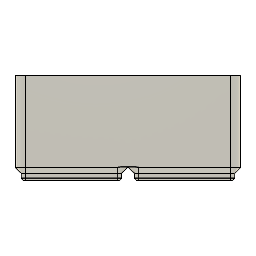
Dupont Jumper Wire (15 cm) (Autodesk Fusion 360 design; units mm, degrees)
Autodesk Fusion 360 part; units mm, degrees
(part 1 of 2)
ref_plane "WorkPlane1" through (0, 0, 0) normal (0, 0, 1) x (1, 0, 0) in component "Gridfinity bin 5x2x5"
sketch "Base plate sketch" plane through (0, 0, 0) normal (0, 0, 1) x (1, 0, 0) in component "Gridfinity bin 5x2x5"
  line L0 (-0.25, -0.25) -> (41.75, -0.25)
  line L1 (41.75, -0.25) -> (41.75, 41.75)
  line L2 (41.75, 41.75) -> (-0.25, 41.75)
  line L3 (-0.25, 41.75) -> (-0.25, -0.25)
  dimension "d326" = 0.25
  dimension "d327" = 0.25
  dimension "d328" = 42
  dimension "d329" = 42
  constraint horizontal L0
  constraint vertical L1
  constraint horizontal L2
  constraint vertical L3
  measures "d326" vertical distance of origin L0.start
  measures "d327" horizontal distance of origin L2.end
  measures "d328" horizontal distance of L0.start L0.end
  measures "d329" vertical distance of L0.end L1.end
extrude "Base top section extrude" add sketch "Base plate sketch" against normal blind 2.4 makes body 1 in component "Gridfinity bin 5x2x5"
fillet "Base corner fillet" radius 4 8 edges at (-0.25, -0.25, -1.2) (41.75, -0.25, -1.2) (41.75, -0.25, -1.2) (41.75, 41.75, -1.2) (41.75, 41.75, -1.2) (-0.25, 41.75, -1.2) (-0.25, 41.75, -1.2) (-0.25, -0.25, -1.2) on bodies 1 in component "Gridfinity bin 5x2x5"
chamfer "Chamfer1" distance 2.4 angle 45 8 edges at (0.9216, 40.5784, -2.4) (-0.25, 20.75, -2.4) (0.9216, 0.9216, -2.4) (20.75, -0.25, -2.4) (40.5784, 0.9216, -2.4) (41.75, 20.75, -2.4) (40.5784, 40.5784, -2.4) (20.75, 41.75, -2.4) on bodies 1 in component "Gridfinity bin 5x2x5"
extrude "Extrude2" add 1 faces at (15.6168, 15.0833, -2.4) along direction (0, 0, -1) blind 2.6 on bodies 1 bodies 1 in component "Gridfinity bin 5x2x5"
chamfer "Chamfer2" distance 0.8 angle 45 8 edges at (2.6186, 38.8814, -5) (20.75, 39.35, -5) (38.8814, 38.8814, -5) (39.35, 20.75, -5) (38.8814, 2.6186, -5) (20.75, 2.15, -5) (2.6186, 2.6186, -5) (2.15, 20.75, -5) on bodies 1 in component "Gridfinity bin 5x2x5"
pattern_linear "R-Pattern1" count 2 spacing 42 along (1, 0, 0) count 5 spacing 42 along (0, 1, 0) of bodies 1 makes body 2 at (68.4167, 16.4167, 0) makes body 3 at (26.4167, 55.75, 0) makes body 4 at (54.4167, 55.75, 0) makes body 5 at (26.4167, 97.75, 0) makes body 6 at (54.4167, 97.75, 0) makes body 7 at (26.4167, 139.75, 0) makes body 8 at (69.75, 141.0833, 0) makes body 9 at (26.4167, 181.75, 0) makes body 10 at (69.75, 183.0833, 0) in component "Gridfinity bin 5x2x5"
sketch "Simple box sketch" plane through (0, 0, 0) normal (0, 0, 1) x (1, 0, 0) in component "Gridfinity bin 5x2x5"
  line L0 (0, 0) -> (83.5, 0)
  line L1 (83.5, 0) -> (83.5, 209.5)
  line L2 (83.5, 209.5) -> (0, 209.5)
  line L3 (0, 209.5) -> (0, 0)
  dimension "d342" = 83.5
  dimension "d343" = 209.5
  constraint horizontal L0
  constraint vertical L1
  constraint horizontal L2
  constraint vertical L3
  constraint coincident L0.start L3
  constraint coincident L3.end L0
  measures "d342" horizontal distance of L0.start L0.end
  measures "d343" vertical distance of L0.end L1.end
extrude "Simple box extrude" add sketch "Simple box sketch" along normal blind 30 separate body makes body 11 in component "Gridfinity bin 5x2x5"
fillet "Bin body corner fillets" radius 3.75 8 edges at (0, 209.5, 15) (83.5, 209.5, 15) (83.5, 209.5, 15) (83.5, 0, 15) (83.5, 0, 15) (0, 0, 15) (0, 0, 15) (0, 209.5, 15) on bodies 11 in component "Gridfinity bin 5x2x5"
ref_plane "WorkPlane2" through (0, 0, 30) normal (0, 0, 1) x (1, 0, 0) in component "Gridfinity bin 5x2x5"
sketch "Simple box at point sketch" plane through (0, 0, 30) normal (0, 0, 1) x (1, 0, 0) in component "Gridfinity bin 5x2x5"
  line L0 (0, 0) -> (83.5, 0)
  line L1 (83.5, 0) -> (83.5, 209.5)
  line L2 (83.5, 209.5) -> (0, 209.5)
  line L3 (0, 209.5) -> (0, 0)
  dimension "d349" = 83.5
  dimension "d350" = 209.5
  constraint horizontal L0
  constraint vertical L1
  constraint horizontal L2
  constraint vertical L3
  constraint coincident L0.start L3
  constraint coincident L3.end L0
  measures "d349" horizontal distance of L0.start L0.end
  measures "d350" vertical distance of L0.end L1.end
extrude "Simple box at point extrude" add sketch "Simple box at point sketch" along normal blind 4.4 separate body makes body 12 in component "Gridfinity bin 5x2x5"
fillet "Lip body corner fillets" radius 3.75 8 edges at (0, 209.5, 32.2) (83.5, 209.5, 32.2) (83.5, 209.5, 32.2) (83.5, 0, 32.2) (83.5, 0, 32.2) (0, 0, 32.2) (0, 0, 32.2) (0, 209.5, 32.2) on bodies 12 in component "Gridfinity bin 5x2x5"
ref_plane "WorkPlane3" through (0, 0, 35) normal (0, 0, 1) x (1, 0, 0) in component "Gridfinity bin 5x2x5"
sketch "Base plate sketch (1)" plane through (0, 0, 35) normal (0, 0, 1) x (1, 0, 0) in component "Gridfinity bin 5x2x5"
  line L0 (-0.5, -0.5) -> (84, -0.5)
  line L1 (84, -0.5) -> (84, 210)
  line L2 (84, 210) -> (-0.5, 210)
  line L3 (-0.5, 210) -> (-0.5, -0.5)
  dimension "d356" = 0.5
  dimension "d357" = 0.5
  dimension "d358" = 84.5
  dimension "d359" = 210.5
  constraint horizontal L0
  constraint vertical L1
  constraint horizontal L2
  constraint vertical L3
  measures "d356" vertical distance of origin L0.start
  measures "d357" horizontal distance of origin L2.end
  measures "d358" horizontal distance of L0.start L0.end
  measures "d359" vertical distance of L0.end L1.end
extrude "Base top section extrude (1)" add sketch "Base plate sketch (1)" against normal blind 2.4 separate body makes body 13 in component "Gridfinity bin 5x2x5"
fillet "Base corner fillet (1)" radius 4.25 8 edges at (-0.5, -0.5, 33.8) (84, -0.5, 33.8) (84, -0.5, 33.8) (84, 210, 33.8) (84, 210, 33.8) (-0.5, 210, 33.8) (-0.5, 210, 33.8) (-0.5, -0.5, 33.8) on bodies 13 in component "Gridfinity bin 5x2x5"
chamfer "Chamfer3" distance 2.4 angle 45 8 edges at (0.7448, 208.7552, 32.6) (-0.5, 104.75, 32.6) (0.7448, 0.7448, 32.6) (41.75, -0.5, 32.6) (82.7552, 0.7448, 32.6) (84, 104.75, 32.6) (82.7552, 208.7552, 32.6) (41.75, 210, 32.6) on bodies 13 in component "Gridfinity bin 5x2x5"
extrude "Extrude6" add 1 faces at (28.4665, 71.0833, 32.6) along direction (0, 0, -1) blind 2.6 on bodies 13 bodies 13 in component "Gridfinity bin 5x2x5"
ref_plane "WorkPlane4" through (41.75, 104.75, 34.4) normal (0, 0, 1) x (1, 0, 0) in component "Gridfinity bin 5x2x5"
sketch "Lip top chamfer" plane through (0, 0, 34.4) normal (0, 0, 1) x (1, 0, 0) in component "Gridfinity bin 5x2x5"
  line L0 (0, 0) -> (83.5, 0)
  line L1 (83.5, 0) -> (83.5, 209.5)
  line L2 (83.5, 209.5) -> (0, 209.5)
  line L3 (0, 209.5) -> (0, 0)
  dimension "d368" = 83.5
  dimension "d369" = 209.5
  constraint horizontal L0
  constraint vertical L1
  constraint horizontal L2
  constraint vertical L3
  constraint coincident L0.start L3
  constraint coincident L3.end L0
  measures "d368" horizontal distance of L0.start L0.end
  measures "d369" vertical distance of L0.end L1.end
extrude "Lip top chamfer cut" add sketch "Lip top chamfer" against normal blind 0.6 separate body makes body 14 in component "Gridfinity bin 5x2x5"
combine "Combine1" operation cut target body 12 tool bodies 14 13 in component "Gridfinity bin 5x2x5"
ref_plane "WorkPlane5" through (0, 0, 30) normal (0, 0, 1) x (1, 0, 0) in component "Gridfinity bin 5x2x5"
sketch "Simple box at point sketch (1)" plane through (0, 0, 30) normal (0, 0, 1) x (1, 0, 0) in component "Gridfinity bin 5x2x5"
  line L0 (1.2, 1.2) -> (82.3, 1.2)
  line L1 (82.3, 1.2) -> (82.3, 208.3)
  line L2 (82.3, 208.3) -> (1.2, 208.3)
  line L3 (1.2, 208.3) -> (1.2, 1.2)
  dimension "d373" = 1.2
  dimension "d374" = 1.2
  dimension "d375" = 81.1
  dimension "d376" = 207.1
  constraint horizontal L0
  constraint vertical L1
  constraint horizontal L2
  constraint vertical L3
  measures "d373" vertical distance of origin L0.start
  measures "d374" horizontal distance of origin L2.end
  measures "d375" horizontal distance of L0.start L0.end
  measures "d376" vertical distance of L0.end L1.end
extrude "Lip bottom chamfer extrude" add sketch "Simple box at point sketch (1)" along normal blind 2.55 separate body makes body 15 in component "Gridfinity bin 5x2x5"
fillet "Fillet5" radius 2.55 8 edges at (1.2, 208.3, 31.275) (82.3, 208.3, 31.275) (82.3, 208.3, 31.275) (82.3, 1.2, 31.275) (82.3, 1.2, 31.275) (1.2, 1.2, 31.275) (1.2, 1.2, 31.275) (1.2, 208.3, 31.275) on bodies 15 in component "Gridfinity bin 5x2x5"
chamfer "Chamfer4" distance 2.55 angle 45 8 edges at (1.9469, 1.9469, 32.55) (41.75, 1.2, 32.55) (81.5531, 1.9469, 32.55) (82.3, 104.75, 32.55) (81.5531, 207.5531, 32.55) (41.75, 208.3, 32.55) (1.9469, 207.5531, 32.55) (1.2, 104.75, 32.55) on bodies 15 in component "Gridfinity bin 5x2x5"
combine "Combine2" operation cut target body 12 tool bodies 15 in component "Gridfinity bin 5x2x5"
ref_plane "WorkPlane6" through (0, 0, 30) normal (0, 0, 1) x (1, 0, 0) in component "Gridfinity bin 5x2x5"
sketch "Inner cutout sketch" plane through (0, 0, 30) normal (0, 0, 1) x (1, 0, 0) in component "Gridfinity bin 5x2x5"
  line L0 (1.2, 1.2) -> (82.3, 1.2)
  line L1 (82.3, 1.2) -> (82.3, 208.3)
  line L2 (82.3, 208.3) -> (1.2, 208.3)
  line L3 (1.2, 208.3) -> (1.2, 1.2)
  dimension "d383" = 1.2
  dimension "d384" = 1.2
  dimension "d385" = 81.1
  dimension "d386" = 207.1
  constraint horizontal L0
  constraint vertical L1
  constraint horizontal L2
  constraint vertical L3
  measures "d383" vertical distance of origin L0.start
  measures "d384" horizontal distance of origin L2.end
  measures "d385" horizontal distance of L0.start L0.end
  measures "d386" vertical distance of L0.end L1.end
extrude "Inner cutout extrude" add sketch "Inner cutout sketch" against normal blind 29 separate body makes body 16 in component "Gridfinity bin 5x2x5"
fillet "Fillet6" radius 2.55 8 edges at (1.2, 1.2, 15.5) (82.3, 1.2, 15.5) (82.3, 1.2, 15.5) (82.3, 208.3, 15.5) (82.3, 208.3, 15.5) (1.2, 208.3, 15.5) (1.2, 208.3, 15.5) (1.2, 1.2, 15.5) on bodies 16 in component "Gridfinity bin 5x2x5"
fillet "Fillet7" radius 2.55 8 edges at (41.75, 208.3, 1) (81.5531, 207.5531, 1) (82.3, 104.75, 1) (81.5531, 1.9469, 1) (41.75, 1.2, 1) (1.9469, 1.9469, 1) (1.2, 104.75, 1) (1.9469, 207.5531, 1) on bodies 16 in component "Gridfinity bin 5x2x5"
combine "Combine3" operation cut target body 11 tool bodies 16 in component "Gridfinity bin 5x2x5"
combine "Combine4" operation add target body 11 tool bodies 12 in component "Gridfinity bin 5x2x5"
ref_plane "WorkPlane7" through (0, 0, 0) normal (0, 0, 1) x (1, 0, 0) in component "Gridfinity bin 5x2x5"
sketch "Base clearance cut sketch" plane through (0, 0, 0) normal (0, 0, 1) x (1, 0, 0) in component "Gridfinity bin 5x2x5"
  line L0 (3.75, 0) -> (79.75, 0)
  line L1 (83.5, 3.75) -> (83.5, 205.75)
  line L2 (79.75, 209.5) -> (3.75, 209.5)
  line L3 (0, 205.75) -> (0, 3.75)
  arc A0 (79.75, 0) -> (83.5, 3.75) centre (79.75, 3.75) ccw
  arc A1 (83.5, 205.75) -> (79.75, 209.5) centre (79.75, 205.75) ccw
  arc A2 (3.75, 209.5) -> (0, 205.75) centre (3.75, 205.75) ccw
  arc A3 (0, 3.75) -> (3.75, 0) centre (3.75, 3.75) ccw
  arc A4 (79.75, -10) -> (93.5, 3.75) centre (79.75, 3.75) ccw
  line L4 (93.5, 3.75) -> (93.5, 205.75)
  arc A5 (93.5, 205.75) -> (79.75, 219.5) centre (79.75, 205.75) ccw
  line L5 (79.75, 219.5) -> (3.75, 219.5)
  arc A6 (3.75, 219.5) -> (-10, 205.75) centre (3.75, 205.75) ccw
  line L6 (-10, 205.75) -> (-10, 3.75)
  arc A7 (-10, 3.75) -> (3.75, -10) centre (3.75, 3.75) ccw
  line L7 (3.75, -10) -> (79.75, -10)
  point P0 (83.5, 0)
  point P1 (83.5, 209.5)
  dimension "d394" = 83.5
  dimension "d395" = 209.5
  dimension "d396" = 3.75
  dimension "d397" = 10
  constraint horizontal L0
  constraint vertical L1
  constraint horizontal L2
  constraint vertical L3
  constraint coincident origin L3
  constraint coincident origin L0
  constraint coincident P0 L0
  constraint coincident P0 L1
  constraint tangent L0 A0
  constraint tangent L1 A0
  constraint coincident P1 L1
  constraint coincident P1 L2
  constraint tangent L1 A1
  constraint tangent L2 A1
  constraint tangent L2 A2
  constraint tangent L3 A2
  constraint tangent L3 A3
  constraint tangent L0 A3
  constraint equal A0 A1
  constraint equal A1 A2
  constraint equal A2 A3
  measures "d394" horizontal distance of origin P0
  measures "d395" vertical distance of P0 P1
  measures "d396" radius of A0
extrude "Base side clearance cut" cut sketch "Base clearance cut sketch" along normal blind 1000 and the other way blind 1000 bodies 1 2 3 4 5 6 7 8 9 10 11 in component "Gridfinity bin 5x2x5"
combine "Combine5" operation add target body 11 tool bodies 2 3 4 5 6 7 8 9 10 1 1 in component "Gridfinity bin 5x2x5"
ref_plane "WorkPlane8" through (41.75, 34.75, 16.775) normal (0, 1, 0) x (1, 0, 0) in component "Gridfinity bin 5x2x5"
ref_plane "WorkPlane9" through (41.75, 174.75, 16.775) normal (0, -1, 0) x (-1, 0, 0) in component "Gridfinity bin 5x2x5"
sketch "Sketch1" plane through (0, 174.75, 0) normal (0, -1, 0) x (-1, 0, 0) in component "Gridfinity bin 5x2x5"
  line L0 (-4.7286, -0.6441) -> (-6.7286, -0.6441)
  line L1 (-4.7286, -23.3407) -> (-4.7286, -0.6441)
  spline S0 degree 5 poles (-4.7286, -23.3407) (-4.8303, -23.4894) (-5.0114, -23.8005) (-5.2163, -24.3082) (-5.3645, -25.0609) (-5.3431, -26.1215) (-5.1246, -27.0811) (-4.8097, -27.882) (-4.5235, -28.4567) (-4.3613, -28.7543) knots 0 0 0 0 0 0 0.2 0.4 0.6 0.8 1 1 1 1 1 1
  line L2 (-4.4864, -22.9867) -> (-4.9707, -23.6947)
  line L3 (-4.7702, -28.0041) -> (-3.9525, -29.5045)
  arc A0 (-4.3613, -28.7543) -> (-3.0333, -28.7553) centre (-3.697, -28.3922) ccw
  spline S1 degree 5 poles (-2.7286, -23.2816) (-2.622, -23.4303) (-2.4314, -23.7419) (-2.2126, -24.252) (-2.0468, -25.0107) (-2.0506, -26.083) (-2.2621, -27.0555) (-2.5781, -27.8686) (-2.8683, -28.4527) (-3.0333, -28.7553) knots 0 0 0 0 0 0 0.2 0.4 0.6 0.8 1 1 1 1 1 1
  line L4 (-2.981, -22.9292) -> (-2.4762, -23.6339)
  line L5 (-2.6192, -27.9959) -> (-3.4475, -29.5147)
  line L6 (-2.7256, -0.5441) -> (-2.7286, -23.2816)
  line L7 (-2.7256, -0.5441) -> (-80.7286, -0.5441)
  line L8 (-80.7286, -0.6441) -> (-80.7286, -0.5441)
  line L9 (-80.7286, -0.6441) -> (-80.7286, -23.2816)
  spline S2 degree 5 poles (-80.7286, -23.2816) (-80.8352, -23.4303) (-81.0256, -23.7421) (-81.2434, -24.2522) (-81.4066, -25.0109) (-81.3989, -26.0829) (-81.1848, -27.055) (-80.868, -27.8678) (-80.5776, -28.4516) (-80.4127, -28.754) knots 0 0 0 0 0 0 0.2 0.4 0.6 0.8 1 1 1 1 1 1
  line L10 (-80.4761, -22.9292) -> (-80.981, -23.6339)
  line L11 (-80.8268, -27.9946) -> (-79.9985, -29.5134)
  arc A1 (-80.4127, -28.754) -> (-79.0957, -28.7539) centre (-79.7542, -28.3949) ccw
  spline S3 degree 5 poles (-78.7286, -23.3407) (-78.6269, -23.4894) (-78.4457, -23.8005) (-78.2409, -24.3081) (-78.0927, -25.0608) (-78.114, -26.1213) (-78.3325, -27.0808) (-78.6473, -27.8816) (-78.9335, -28.4563) (-79.0957, -28.7539) knots 0 0 0 0 0 0 0.2 0.4 0.6 0.8 1 1 1 1 1 1
  line L12 (-78.9707, -22.9867) -> (-78.4864, -23.6947)
  line L13 (-78.6868, -28.0037) -> (-79.5046, -29.504)
  line L14 (-78.7286, -23.3407) -> (-78.7286, -0.6441)
  line L15 (-78.7286, -0.6441) -> (-76.7286, -0.6441)
  line L16 (-76.7286, -0.6441) -> (-76.7286, -23.2816)
  spline S4 degree 5 poles (-76.7286, -23.2816) (-76.8353, -23.4305) (-77.0257, -23.7426) (-77.2426, -24.2531) (-77.4032, -25.0122) (-77.3913, -26.0846) (-77.1743, -27.0569) (-76.8559, -27.8697) (-76.565, -28.4535) (-76.3999, -28.7559) knots 0 0 0 0 0 0 0.2 0.4 0.6 0.8 1 1 1 1 1 1
  line L17 (-76.4761, -22.9292) -> (-76.981, -23.6339)
  line L18 (-76.8145, -27.9967) -> (-75.9854, -29.5151)
  arc A2 (-76.3999, -28.7559) -> (-75.0957, -28.7539) centre (-75.7484, -28.3981) ccw
  spline S5 degree 5 poles (-74.7286, -23.3407) (-74.6269, -23.4894) (-74.4457, -23.8005) (-74.2409, -24.3081) (-74.0927, -25.0608) (-74.114, -26.1213) (-74.3325, -27.0808) (-74.6473, -27.8816) (-74.9335, -28.4563) (-75.0957, -28.7539) knots 0 0 0 0 0 0 0.2 0.4 0.6 0.8 1 1 1 1 1 1
  line L19 (-74.9707, -22.9867) -> (-74.4864, -23.6947)
  line L20 (-74.6868, -28.0037) -> (-75.5046, -29.504)
  line L21 (-74.7286, -23.3407) -> (-74.7286, -0.6441)
  line L22 (-74.7286, -0.6441) -> (-72.7286, -0.6441)
  line L23 (-72.7286, -0.6441) -> (-72.7286, -23.2816)
  spline S6 degree 5 poles (-72.7286, -23.2816) (-72.8352, -23.4303) (-73.0256, -23.7421) (-73.2434, -24.2522) (-73.4066, -25.0109) (-73.3989, -26.0829) (-73.1848, -27.0551) (-72.8679, -27.8678) (-72.5776, -28.4516) (-72.4127, -28.754) knots 0 0 0 0 0 0 0.2 0.4 0.6 0.8 1 1 1 1 1 1
  line L24 (-72.4761, -22.9292) -> (-72.981, -23.6339)
  line L25 (-72.8268, -27.9947) -> (-71.9985, -29.5134)
  arc A3 (-72.4127, -28.754) -> (-71.0957, -28.7539) centre (-71.7542, -28.3949) ccw
  spline S7 degree 5 poles (-70.7286, -23.3407) (-70.6269, -23.4894) (-70.4457, -23.8005) (-70.2409, -24.3081) (-70.0927, -25.0608) (-70.114, -26.1213) (-70.3325, -27.0808) (-70.6473, -27.8816) (-70.9335, -28.4563) (-71.0957, -28.7539) knots 0 0 0 0 0 0 0.2 0.4 0.6 0.8 1 1 1 1 1 1
  line L26 (-70.9707, -22.9867) -> (-70.4864, -23.6947)
  line L27 (-70.6868, -28.0037) -> (-71.5046, -29.504)
  line L28 (-70.7286, -23.3407) -> (-70.7286, -0.6441)
  line L29 (-68.7286, -0.6441) -> (-70.7286, -0.6441)
  line L30 (-68.7286, -23.3407) -> (-68.7286, -0.6441)
  spline S8 degree 5 poles (-68.7286, -23.3407) (-68.8303, -23.4894) (-69.0114, -23.8005) (-69.2162, -24.3081) (-69.3644, -25.0608) (-69.3431, -26.1213) (-69.1247, -27.0808) (-68.8098, -27.8816) (-68.5236, -28.4563) (-68.3614, -28.7539) knots 0 0 0 0 0 0 0.2 0.4 0.6 0.8 1 1 1 1 1 1
  line L31 (-68.4864, -22.9867) -> (-68.9707, -23.6947)
  line L32 (-68.7703, -28.0037) -> (-67.9526, -29.504)
  arc A4 (-68.3614, -28.7539) -> (-67.0445, -28.754) centre (-67.7029, -28.3949) ccw
  spline S9 degree 5 poles (-66.7286, -23.2816) (-66.622, -23.4303) (-66.4315, -23.7421) (-66.2137, -24.2522) (-66.0506, -25.0109) (-66.0583, -26.0829) (-66.2723, -27.055) (-66.5892, -27.8678) (-66.8795, -28.4516) (-67.0445, -28.754) knots 0 0 0 0 0 0 0.2 0.4 0.6 0.8 1 1 1 1 1 1
  line L33 (-66.981, -22.9292) -> (-66.4762, -23.6339)
  line L34 (-66.6303, -27.9946) -> (-67.4586, -29.5134)
  line L35 (-66.7286, -0.6441) -> (-66.7286, -23.2816)
  line L36 (-64.7286, -0.6441) -> (-66.7286, -0.6441)
  line L37 (-64.7286, -23.3407) -> (-64.7286, -0.6441)
  spline S10 degree 5 poles (-64.7286, -23.3407) (-64.8303, -23.4894) (-65.0114, -23.8005) (-65.2162, -24.3081) (-65.3644, -25.0608) (-65.3431, -26.1213) (-65.1247, -27.0808) (-64.8098, -27.8816) (-64.5236, -28.4563) (-64.3614, -28.7539) knots 0 0 0 0 0 0 0.2 0.4 0.6 0.8 1 1 1 1 1 1
  line L38 (-64.4864, -22.9867) -> (-64.9707, -23.6947)
  line L39 (-64.7703, -28.0037) -> (-63.9526, -29.504)
  arc A5 (-64.3614, -28.7539) -> (-63.0572, -28.7559) centre (-63.7088, -28.3981) ccw
  spline S11 degree 5 poles (-62.7286, -23.2816) (-62.6219, -23.4305) (-62.4314, -23.7426) (-62.2146, -24.2531) (-62.0539, -25.0122) (-62.0658, -26.0846) (-62.2829, -27.0569) (-62.6012, -27.8697) (-62.8921, -28.4535) (-63.0572, -28.7559) knots 0 0 0 0 0 0 0.2 0.4 0.6 0.8 1 1 1 1 1 1
  line L40 (-62.981, -22.9292) -> (-62.4762, -23.6339)
  line L41 (-62.6427, -27.9967) -> (-63.4718, -29.5151)
  line L42 (-62.7286, -0.6441) -> (-62.7286, -23.2816)
  line L43 (-60.7286, -0.6441) -> (-62.7286, -0.6441)
  line L44 (-60.7286, -23.3407) -> (-60.7286, -0.6441)
  spline S12 degree 5 poles (-60.7286, -23.3407) (-60.8303, -23.4894) (-61.0114, -23.8005) (-61.2162, -24.3081) (-61.3644, -25.0608) (-61.3431, -26.1213) (-61.1247, -27.0808) (-60.8098, -27.8816) (-60.5236, -28.4563) (-60.3614, -28.7539) knots 0 0 0 0 0 0 0.2 0.4 0.6 0.8 1 1 1 1 1 1
  line L45 (-60.4864, -22.9867) -> (-60.9707, -23.6947)
  line L46 (-60.7703, -28.0037) -> (-59.9526, -29.504)
  arc A6 (-60.3614, -28.7539) -> (-59.0445, -28.754) centre (-59.7029, -28.3949) ccw
  spline S13 degree 5 poles (-58.7286, -23.2816) (-58.622, -23.4303) (-58.4315, -23.7421) (-58.2137, -24.2522) (-58.0505, -25.0109) (-58.0583, -26.0829) (-58.2723, -27.055) (-58.5892, -27.8678) (-58.8795, -28.4516) (-59.0445, -28.754) knots 0 0 0 0 0 0 0.2 0.4 0.6 0.8 1 1 1 1 1 1
  line L47 (-58.981, -22.9292) -> (-58.4762, -23.6339)
  line L48 (-58.6303, -27.9946) -> (-59.4586, -29.5134)
  line L49 (-58.7286, -0.6441) -> (-58.7286, -23.2816)
  line L50 (-56.7286, -0.6441) -> (-58.7286, -0.6441)
  line L51 (-56.7286, -23.3407) -> (-56.7286, -0.6441)
  spline S14 degree 5 poles (-56.7286, -23.3407) (-56.8308, -23.4902) (-57.0136, -23.8029) (-57.2231, -24.3136) (-57.3808, -25.0714) (-57.3723, -26.1397) (-57.1608, -27.1068) (-56.8471, -27.9141) (-56.5595, -28.4935) (-56.396, -28.7936) knots 0 0 0 0 0 0 0.2 0.4 0.6 0.8 1 1 1 1 1 1
  line L52 (-56.4864, -22.9867) -> (-56.9707, -23.6947)
  line L53 (-56.8047, -28.0433) -> (-55.9873, -29.5438)
  arc A7 (-56.396, -28.7936) -> (-55.0632, -28.7994) centre (-55.728, -28.4296) ccw
  spline S15 degree 5 poles (-54.7286, -23.2816) (-54.621, -23.4317) (-54.4279, -23.7467) (-54.2042, -24.2631) (-54.0305, -25.0323) (-54.0294, -26.1179) (-54.2483, -27.0981) (-54.581, -27.9135) (-54.8882, -28.4974) (-55.0632, -28.7994) knots 0 0 0 0 0 0 0.2 0.4 0.6 0.8 1 1 1 1 1 1
  line L54 (-54.981, -22.9292) -> (-54.4762, -23.6339)
  line L55 (-54.6296, -28.051) -> (-55.4968, -29.5477)
  line L56 (-54.7286, -0.6441) -> (-54.7286, -23.2816)
  line L57 (-52.7286, -0.6441) -> (-54.7286, -0.6441)
  line L58 (-52.7286, -23.3407) -> (-52.7286, -0.6441)
  spline S16 degree 5 poles (-52.7286, -23.3407) (-52.8303, -23.4894) (-53.0114, -23.8005) (-53.2163, -24.3082) (-53.3645, -25.0609) (-53.3431, -26.1215) (-53.1246, -27.0811) (-52.8097, -27.882) (-52.5235, -28.4567) (-52.3613, -28.7543) knots 0 0 0 0 0 0 0.2 0.4 0.6 0.8 1 1 1 1 1 1
  line L59 (-52.4864, -22.9867) -> (-52.9707, -23.6947)
  line L60 (-52.7702, -28.0041) -> (-51.9525, -29.5045)
  arc A8 (-52.3613, -28.7543) -> (-51.0333, -28.7553) centre (-51.697, -28.3922) ccw
  spline S17 degree 5 poles (-50.7286, -23.2816) (-50.622, -23.4303) (-50.4314, -23.7419) (-50.2126, -24.252) (-50.0468, -25.0107) (-50.0506, -26.083) (-50.2621, -27.0555) (-50.5781, -27.8686) (-50.8683, -28.4527) (-51.0333, -28.7553) knots 0 0 0 0 0 0 0.2 0.4 0.6 0.8 1 1 1 1 1 1
  line L61 (-50.981, -22.9292) -> (-50.4762, -23.6339)
  line L62 (-50.6192, -27.9959) -> (-51.4475, -29.5147)
  line L63 (-50.7286, -0.6441) -> (-50.7286, -23.2816)
  line L64 (-48.7286, -0.6441) -> (-50.7286, -0.6441)
  line L65 (-48.7286, -0.6441) -> (-48.7286, -23.2816)
  spline S18 degree 5 poles (-48.7286, -23.2816) (-48.8349, -23.43) (-49.0265, -23.7414) (-49.2509, -24.2523) (-49.4303, -25.0138) (-49.4431, -26.0891) (-49.2338, -27.0603) (-48.9072, -27.8685) (-48.6034, -28.4473) (-48.4299, -28.7467) knots 0 0 0 0 0 0 0.2 0.4 0.6 0.8 1 1 1 1 1 1
  line L66 (-48.4762, -22.9292) -> (-48.981, -23.6339)
  line L67 (-48.8635, -27.9984) -> (-47.9963, -29.495)
  arc A9 (-48.4299, -28.7467) -> (-47.0769, -28.7466) centre (-47.7534, -28.3567) ccw
  spline S19 degree 5 poles (-46.7286, -23.3407) (-46.6271, -23.489) (-46.4448, -23.7998) (-46.2333, -24.3082) (-46.0686, -25.0637) (-46.069, -26.1275) (-46.2824, -27.0861) (-46.6067, -27.8824) (-46.9062, -28.4521) (-47.0769, -28.7466) knots 0 0 0 0 0 0 0.2 0.4 0.6 0.8 1 1 1 1 1 1
  line L68 (-46.9707, -22.9867) -> (-46.4864, -23.6947)
  line L69 (-46.6486, -28.0074) -> (-47.5052, -29.4857)
  line L70 (-46.7286, -23.3407) -> (-46.7286, -0.6441)
  line L71 (-46.7286, -0.6441) -> (-44.7286, -0.6441)
  line L72 (-44.7286, -0.6441) -> (-44.7286, -23.2816)
  spline S20 degree 5 poles (-44.7286, -23.2816) (-44.8351, -23.4303) (-45.0258, -23.7419) (-45.2445, -24.252) (-45.4104, -25.0107) (-45.4066, -26.083) (-45.1952, -27.0555) (-44.8792, -27.8686) (-44.589, -28.4528) (-44.424, -28.7554) knots 0 0 0 0 0 0 0.2 0.4 0.6 0.8 1 1 1 1 1 1
  line L73 (-44.4761, -22.9292) -> (-44.981, -23.6339)
  line L74 (-44.8381, -27.996) -> (-44.0098, -29.5147)
  arc A10 (-44.424, -28.7554) -> (-43.0957, -28.7539) centre (-43.7602, -28.3928) ccw
  spline S21 degree 5 poles (-42.7286, -23.3407) (-42.6269, -23.4894) (-42.4457, -23.8005) (-42.2409, -24.3081) (-42.0927, -25.0608) (-42.114, -26.1213) (-42.3325, -27.0808) (-42.6473, -27.8816) (-42.9335, -28.4563) (-43.0957, -28.7539) knots 0 0 0 0 0 0 0.2 0.4 0.6 0.8 1 1 1 1 1 1
  line L75 (-42.9707, -22.9867) -> (-42.4864, -23.6947)
  line L76 (-42.6868, -28.0037) -> (-43.5046, -29.504)
  line L77 (-42.7286, -23.3407) -> (-42.7286, -0.6441)
  line L78 (-42.7286, -0.6441) -> (-40.7286, -0.6441)
  line L79 (-40.7286, -0.6441) -> (-40.7286, -23.2816)
  spline S22 degree 5 poles (-40.7286, -23.2816) (-40.8361, -23.4317) (-41.0293, -23.7467) (-41.253, -24.2631) (-41.4266, -25.0323) (-41.4278, -26.1179) (-41.2088, -27.0981) (-40.8762, -27.9135) (-40.569, -28.4974) (-40.394, -28.7994) knots 0 0 0 0 0 0 0.2 0.4 0.6 0.8 1 1 1 1 1 1
  line L80 (-40.4761, -22.9292) -> (-40.981, -23.6339)
  line L81 (-40.8276, -28.051) -> (-39.9604, -29.5477)
  arc A11 (-40.394, -28.7994) -> (-39.0612, -28.7936) centre (-39.7292, -28.4296) ccw
  spline S23 degree 5 poles (-38.7286, -23.3407) (-38.6263, -23.4902) (-38.4435, -23.8029) (-38.234, -24.3136) (-38.0764, -25.0714) (-38.0849, -26.1397) (-38.2963, -27.1068) (-38.61, -27.9141) (-38.8977, -28.4935) (-39.0612, -28.7936) knots 0 0 0 0 0 0 0.2 0.4 0.6 0.8 1 1 1 1 1 1
  line L82 (-38.9707, -22.9867) -> (-38.4864, -23.6947)
  line L83 (-38.6524, -28.0433) -> (-39.4699, -29.5438)
  line L84 (-38.7286, -23.3407) -> (-38.7286, -0.6441)
  line L85 (-38.7286, -0.6441) -> (-36.7286, -0.6441)
  line L86 (-36.7286, -0.6441) -> (-36.7286, -23.2816)
  spline S24 degree 5 poles (-36.7286, -23.2816) (-36.8352, -23.4303) (-37.0256, -23.7421) (-37.2434, -24.2522) (-37.4066, -25.0109) (-37.3989, -26.0829) (-37.1848, -27.055) (-36.868, -27.8678) (-36.5776, -28.4516) (-36.4127, -28.754) knots 0 0 0 0 0 0 0.2 0.4 0.6 0.8 1 1 1 1 1 1
  line L87 (-36.4761, -22.9292) -> (-36.981, -23.6339)
  line L88 (-36.8268, -27.9946) -> (-35.9985, -29.5134)
  arc A12 (-36.4127, -28.754) -> (-35.0957, -28.7539) centre (-35.7542, -28.3949) ccw
  spline S25 degree 5 poles (-34.7286, -23.3407) (-34.6269, -23.4894) (-34.4457, -23.8005) (-34.2409, -24.3081) (-34.0927, -25.0608) (-34.114, -26.1213) (-34.3325, -27.0808) (-34.6473, -27.8816) (-34.9335, -28.4563) (-35.0957, -28.7539) knots 0 0 0 0 0 0 0.2 0.4 0.6 0.8 1 1 1 1 1 1
  line L89 (-34.9707, -22.9867) -> (-34.4864, -23.6947)
  line L90 (-34.6868, -28.0037) -> (-35.5046, -29.504)
  line L91 (-34.7286, -23.3407) -> (-34.7286, -0.6441)
  line L92 (-34.7286, -0.6441) -> (-32.7286, -0.6441)
  line L93 (-32.7286, -0.6441) -> (-32.7286, -23.2816)
  spline S26 degree 5 poles (-32.7286, -23.2816) (-32.8353, -23.4305) (-33.0257, -23.7426) (-33.2426, -24.2531) (-33.4032, -25.0122) (-33.3913, -26.0846) (-33.1743, -27.0569) (-32.8559, -27.8697) (-32.565, -28.4535) (-32.3999, -28.7559) knots 0 0 0 0 0 0 0.2 0.4 0.6 0.8 1 1 1 1 1 1
  line L94 (-32.4761, -22.9292) -> (-32.981, -23.6339)
  line L95 (-32.8145, -27.9967) -> (-31.9854, -29.5151)
  arc A13 (-32.3999, -28.7559) -> (-31.0957, -28.7539) centre (-31.7484, -28.3981) ccw
  spline S27 degree 5 poles (-30.7286, -23.3407) (-30.6269, -23.4894) (-30.4457, -23.8005) (-30.2409, -24.3081) (-30.0927, -25.0608) (-30.114, -26.1213) (-30.3325, -27.0808) (-30.6473, -27.8816) (-30.9335, -28.4563) (-31.0957, -28.7539) knots 0 0 0 0 0 0 0.2 0.4 0.6 0.8 1 1 1 1 1 1
  line L96 (-30.9707, -22.9867) -> (-30.4864, -23.6947)
  line L97 (-30.6868, -28.0037) -> (-31.5046, -29.504)
  line L98 (-30.7286, -23.3407) -> (-30.7286, -0.6441)
  line L99 (-30.7286, -0.6441) -> (-28.7286, -0.6441)
  line L100 (-28.7286, -0.6441) -> (-28.7286, -23.2816)
  spline S28 degree 5 poles (-28.7286, -23.2816) (-28.8352, -23.4303) (-29.0256, -23.7421) (-29.2434, -24.2522) (-29.4066, -25.0109) (-29.3989, -26.0829) (-29.1848, -27.0551) (-28.8679, -27.8678) (-28.5776, -28.4516) (-28.4127, -28.754) knots 0 0 0 0 0 0 0.2 0.4 0.6 0.8 1 1 1 1 1 1
  line L101 (-28.4761, -22.9292) -> (-28.981, -23.6339)
  line L102 (-28.8268, -27.9947) -> (-27.9985, -29.5134)
  arc A14 (-28.4127, -28.754) -> (-27.0957, -28.7539) centre (-27.7542, -28.3949) ccw
  spline S29 degree 5 poles (-26.7286, -23.3407) (-26.6269, -23.4894) (-26.4457, -23.8005) (-26.2409, -24.3081) (-26.0927, -25.0608) (-26.114, -26.1213) (-26.3325, -27.0808) (-26.6473, -27.8816) (-26.9335, -28.4563) (-27.0957, -28.7539) knots 0 0 0 0 0 0 0.2 0.4 0.6 0.8 1 1 1 1 1 1
  line L103 (-26.9707, -22.9867) -> (-26.4864, -23.6947)
  line L104 (-26.6868, -28.0037) -> (-27.5046, -29.504)
  line L105 (-26.7286, -23.3407) -> (-26.7286, -0.6441)
  line L106 (-24.7286, -0.6441) -> (-26.7286, -0.6441)
  line L107 (-24.7286, -23.3407) -> (-24.7286, -0.6441)
  spline S30 degree 5 poles (-24.7286, -23.3407) (-24.8303, -23.4894) (-25.0114, -23.8005) (-25.2162, -24.3081) (-25.3644, -25.0608) (-25.3431, -26.1213) (-25.1247, -27.0808) (-24.8098, -27.8816) (-24.5236, -28.4563) (-24.3614, -28.7539) knots 0 0 0 0 0 0 0.2 0.4 0.6 0.8 1 1 1 1 1 1
  line L108 (-24.4864, -22.9867) -> (-24.9707, -23.6947)
  line L109 (-24.7703, -28.0037) -> (-23.9526, -29.504)
  arc A15 (-24.3614, -28.7539) -> (-23.0445, -28.754) centre (-23.7029, -28.3949) ccw
  spline S31 degree 5 poles (-22.7286, -23.2816) (-22.622, -23.4303) (-22.4315, -23.7421) (-22.2137, -24.2522) (-22.0506, -25.0109) (-22.0583, -26.0829) (-22.2723, -27.055) (-22.5892, -27.8678) (-22.8795, -28.4516) (-23.0445, -28.754) knots 0 0 0 0 0 0 0.2 0.4 0.6 0.8 1 1 1 1 1 1
  line L110 (-22.981, -22.9292) -> (-22.4762, -23.6339)
  line L111 (-22.6303, -27.9946) -> (-23.4586, -29.5134)
  line L112 (-22.7286, -0.6441) -> (-22.7286, -23.2816)
  line L113 (-20.7286, -0.6441) -> (-22.7286, -0.6441)
  line L114 (-20.7286, -23.3407) -> (-20.7286, -0.6441)
  spline S32 degree 5 poles (-20.7286, -23.3407) (-20.8303, -23.4894) (-21.0114, -23.8005) (-21.2162, -24.3081) (-21.3644, -25.0608) (-21.3431, -26.1213) (-21.1247, -27.0808) (-20.8098, -27.8816) (-20.5236, -28.4563) (-20.3614, -28.7539) knots 0 0 0 0 0 0 0.2 0.4 0.6 0.8 1 1 1 1 1 1
  line L115 (-20.4864, -22.9867) -> (-20.9707, -23.6947)
  line L116 (-20.7703, -28.0037) -> (-19.9526, -29.504)
  arc A16 (-20.3614, -28.7539) -> (-19.0572, -28.7559) centre (-19.7088, -28.3981) ccw
  spline S33 degree 5 poles (-18.7286, -23.2816) (-18.6219, -23.4305) (-18.4314, -23.7426) (-18.2146, -24.2531) (-18.0539, -25.0122) (-18.0658, -26.0846) (-18.2829, -27.0569) (-18.6012, -27.8697) (-18.8921, -28.4535) (-19.0572, -28.7559) knots 0 0 0 0 0 0 0.2 0.4 0.6 0.8 1 1 1 1 1 1
  line L117 (-18.981, -22.9292) -> (-18.4762, -23.6339)
  line L118 (-18.6427, -27.9967) -> (-19.4718, -29.5151)
  line L119 (-18.7286, -0.6441) -> (-18.7286, -23.2816)
  line L120 (-16.7286, -0.6441) -> (-18.7286, -0.6441)
  line L121 (-16.7286, -23.3407) -> (-16.7286, -0.6441)
  spline S34 degree 5 poles (-16.7286, -23.3407) (-16.8303, -23.4894) (-17.0114, -23.8005) (-17.2162, -24.3081) (-17.3644, -25.0608) (-17.3431, -26.1213) (-17.1247, -27.0808) (-16.8098, -27.8816) (-16.5236, -28.4563) (-16.3614, -28.7539) knots 0 0 0 0 0 0 0.2 0.4 0.6 0.8 1 1 1 1 1 1
  line L122 (-16.4864, -22.9867) -> (-16.9707, -23.6947)
  line L123 (-16.7703, -28.0037) -> (-15.9526, -29.504)
  arc A17 (-16.3614, -28.7539) -> (-15.0445, -28.754) centre (-15.7029, -28.3949) ccw
  spline S35 degree 5 poles (-14.7286, -23.2816) (-14.622, -23.4303) (-14.4315, -23.7421) (-14.2137, -24.2522) (-14.0505, -25.0109) (-14.0583, -26.0829) (-14.2723, -27.055) (-14.5892, -27.8678) (-14.8795, -28.4516) (-15.0445, -28.754) knots 0 0 0 0 0 0 0.2 0.4 0.6 0.8 1 1 1 1 1 1
  line L124 (-14.981, -22.9292) -> (-14.4762, -23.6339)
  line L125 (-14.6303, -27.9946) -> (-15.4586, -29.5134)
  line L126 (-14.7286, -0.6441) -> (-14.7286, -23.2816)
  line L127 (-12.7286, -0.6441) -> (-14.7286, -0.6441)
  line L128 (-12.7286, -23.3407) -> (-12.7286, -0.6441)
  spline S36 degree 5 poles (-12.7286, -23.3407) (-12.8308, -23.4902) (-13.0136, -23.8029) (-13.2231, -24.3136) (-13.3808, -25.0714) (-13.3723, -26.1397) (-13.1608, -27.1068) (-12.8471, -27.9141) (-12.5595, -28.4935) (-12.396, -28.7936) knots 0 0 0 0 0 0 0.2 0.4 0.6 0.8 1 1 1 1 1 1
  line L129 (-12.4864, -22.9867) -> (-12.9707, -23.6947)
  line L130 (-12.8047, -28.0433) -> (-11.9873, -29.5438)
  arc A18 (-12.396, -28.7936) -> (-11.0632, -28.7994) centre (-11.728, -28.4296) ccw
  spline S37 degree 5 poles (-10.7286, -23.2816) (-10.621, -23.4317) (-10.4279, -23.7467) (-10.2042, -24.2631) (-10.0305, -25.0323) (-10.0294, -26.1179) (-10.2483, -27.0981) (-10.581, -27.9135) (-10.8882, -28.4974) (-11.0632, -28.7994) knots 0 0 0 0 0 0 0.2 0.4 0.6 0.8 1 1 1 1 1 1
  line L131 (-10.981, -22.9292) -> (-10.4762, -23.6339)
  line L132 (-10.6296, -28.051) -> (-11.4968, -29.5477)
  line L133 (-10.7286, -0.6441) -> (-10.7286, -23.2816)
  line L134 (-8.7286, -0.6441) -> (-10.7286, -0.6441)
  line L135 (-8.7286, -23.3407) -> (-8.7286, -0.6441)
  spline S38 degree 5 poles (-8.7286, -23.3407) (-8.8303, -23.4894) (-9.0114, -23.8005) (-9.2163, -24.3082) (-9.3645, -25.0609) (-9.3431, -26.1215) (-9.1246, -27.0811) (-8.8097, -27.882) (-8.5235, -28.4567) (-8.3613, -28.7543) knots 0 0 0 0 0 0 0.2 0.4 0.6 0.8 1 1 1 1 1 1
  line L136 (-8.4864, -22.9867) -> (-8.9707, -23.6947)
  line L137 (-8.7702, -28.0041) -> (-7.9525, -29.5045)
  arc A19 (-8.3613, -28.7543) -> (-7.0333, -28.7553) centre (-7.697, -28.3922) ccw
  spline S39 degree 5 poles (-6.7286, -23.2816) (-6.622, -23.4303) (-6.4314, -23.7419) (-6.2126, -24.252) (-6.0468, -25.0107) (-6.0506, -26.083) (-6.2621, -27.0555) (-6.5781, -27.8686) (-6.8683, -28.4527) (-7.0333, -28.7553) knots 0 0 0 0 0 0 0.2 0.4 0.6 0.8 1 1 1 1 1 1
  line L138 (-6.981, -22.9292) -> (-6.4762, -23.6339)
  line L139 (-6.6192, -27.9959) -> (-7.4475, -29.5147)
  line L140 (-6.7286, -0.6441) -> (-6.7286, -23.2816)
  dimension "d441" = 0.1
  dimension "d442" = 2
  dimension "d443" = 2
  dimension "d444" = 2
  dimension "d445" = 2
  dimension "d446" = 2
  dimension "d447" = 2
  dimension "d448" = 2
  dimension "d449" = 2
  dimension "d450" = 2
  dimension "d451" = 2
  dimension "d452" = 2
  dimension "d453" = 2
  dimension "d454" = 2
  dimension "d455" = 2
  dimension "d456" = 2
  dimension "d457" = 2
  dimension "d458" = 2
  dimension "d459" = 2
  dimension "d460" = 0.1
  dimension "d461" = 0.1
  dimension "d462" = 0.1
  dimension "d463" = 0.1
  dimension "d464" = 0.1
  dimension "d465" = 0.1
  dimension "d466" = 0.1
  dimension "d467" = 0.1
  dimension "d468" = 0.1
  dimension "d469" = 0.1
  dimension "d470" = 0.1
  dimension "d471" = 0.1
  dimension "d472" = 0.1
  dimension "d473" = 0.1
  dimension "d474" = 0.1
  dimension "d475" = 0.1
  dimension "d476" = 0.1
  dimension "d477" = 0.1
  constraint tangent A19 S39
  constraint tangent S38 A19
  constraint midpoint L135.start L136
  constraint midpoint S38.end L137
  constraint midpoint S39.start L138
  constraint midpoint A19.end L139
  constraint tangent S36 A18
  constraint midpoint L128.start L129
  constraint midpoint S36.end L130
  constraint midpoint S37.start L131
  constraint midpoint A18.end L132
  constraint midpoint L121.start L122
  constraint midpoint S34.end L123
  constraint midpoint S35.start L124
  constraint midpoint A17.end L125
  constraint midpoint S33.start L117
  constraint midpoint A16.end L118
  constraint tangent S32 A16
  constraint midpoint L114.start L115
  constraint midpoint S32.end L116
  constraint tangent A15 S31
  constraint tangent S30 A15
  constraint midpoint L107.start L108
  constraint midpoint S30.end L109
  constraint midpoint S31.start L110
  constraint midpoint A15.end L111
  constraint tangent A8 S17
  constraint tangent S16 A8
  constraint midpoint L58.start L59
  constraint midpoint S16.end L60
  constraint midpoint S17.start L61
  constraint midpoint A8.end L62
  constraint tangent S14 A7
  constraint midpoint L51.start L52
  constraint midpoint S14.end L53
  constraint midpoint S15.start L54
  constraint midpoint A7.end L55
  constraint midpoint L44.start L45
  constraint midpoint S12.end L46
  constraint midpoint S13.start L47
  constraint midpoint A6.end L48
  constraint midpoint S11.start L40
  constraint midpoint A5.end L41
  constraint tangent S10 A5
  constraint midpoint L37.start L38
  constraint midpoint S10.end L39
  constraint tangent A4 S9
  constraint tangent S8 A4
  constraint midpoint L30.start L31
  constraint midpoint S8.end L32
  constraint midpoint S9.start L33
  constraint midpoint A4.end L34
  constraint horizontal L64
  constraint horizontal L7
  constraint tangent A0 S1
  constraint tangent S0 A0
  constraint midpoint L1.start L2
  constraint midpoint S0.end L3
  constraint midpoint S1.start L4
  constraint midpoint A0.end L5
  constraint perpendicular L7 L8
  measures "d441" distance of L0 L7
  measures "d442" distance of L133 L135
  measures "d443" distance of L126 L128
  measures "d444" distance of L119 L121
  measures "d445" distance of L112 L114
  measures "d446" distance of L105 L107
  measures "d447" distance of L98 L100
  measures "d448" distance of L91 L93
  measures "d449" distance of L84 L86
  measures "d450" distance of L77 L79
  measures "d451" distance of L70 L72
  measures "d452" distance of L63 L65
  measures "d453" distance of L56 L58
  measures "d454" distance of L49 L51
  measures "d455" distance of L42 L44
  measures "d456" distance of L35 L37
  measures "d457" distance of L28 L30
  measures "d458" distance of L21 L23
  measures "d459" distance of L14 L16
  measures "d460" distance of L7 L134
  measures "d461" distance of L7 L127
  measures "d462" distance of L7 L120
  measures "d463" distance of L7 L113
  measures "d464" distance of L7 L106
  measures "d465" distance of L7 L99
  measures "d466" distance of L7 L92
  measures "d467" distance of L7 L85
  measures "d468" distance of L7 L78
  measures "d469" distance of L7 L71
  measures "d470" distance of L7 L64
  measures "d471" distance of L7 L57
  measures "d472" distance of L7 L50
  measures "d473" distance of L7 L43
  measures "d474" distance of L7 L36
  measures "d475" distance of L7 L29
  measures "d476" distance of L7 L22
  measures "d477" distance of L7 L15